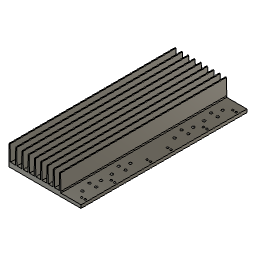
Reproduction Amplifone Deflection Heat Sink (Autodesk Fusion 360 design; units mm, degrees)
Autodesk Fusion 360 part; units mm, degrees
sketch "Sketch1" plane through (0, 0, 0) normal (0, 1, 0) x (1, 0, 0)
  line L0 (-62.23, 0) -> (62.23, 0)
  line L1 (-1.2573, -7.62) -> (1.2573, -7.62) construction
  line L2 (0, -7.62) -> (0, -33.02) construction
  line L3 (-0.762, -33.02) -> (0.762, -33.02)
  line L4 (-1.2573, -7.62) -> (-0.762, -33.02)
  line L5 (1.2573, -7.62) -> (0.762, -33.02)
  line L6 (-51.562, -33.02) -> (-50.038, -33.02)
  line L7 (-49.5427, -7.62) -> (-50.038, -33.02)
  line L8 (-52.0573, -7.62) -> (-51.562, -33.02)
  line L9 (-52.0573, -7.62) -> (-49.5427, -7.62) construction
  line L10 (-50.8, -7.62) -> (-50.8, -33.02) construction
  line L11 (-41.402, -33.02) -> (-39.878, -33.02)
  line L12 (-39.3827, -7.62) -> (-39.878, -33.02)
  line L13 (-41.8973, -7.62) -> (-41.402, -33.02)
  line L14 (-41.8973, -7.62) -> (-39.3827, -7.62) construction
  line L15 (-40.64, -7.62) -> (-40.64, -33.02) construction
  line L16 (-31.242, -33.02) -> (-29.718, -33.02)
  line L17 (-29.2227, -7.62) -> (-29.718, -33.02)
  line L18 (-31.7373, -7.62) -> (-31.242, -33.02)
  line L19 (-31.7373, -7.62) -> (-29.2227, -7.62) construction
  line L20 (-30.48, -7.62) -> (-30.48, -33.02) construction
  line L21 (-21.082, -33.02) -> (-19.558, -33.02)
  line L22 (-19.0627, -7.62) -> (-19.558, -33.02)
  line L23 (-21.5773, -7.62) -> (-21.082, -33.02)
  line L24 (-21.5773, -7.62) -> (-19.0627, -7.62) construction
  line L25 (-20.32, -7.62) -> (-20.32, -33.02) construction
  line L26 (-10.922, -33.02) -> (-9.398, -33.02)
  line L27 (-8.9027, -7.62) -> (-9.398, -33.02)
  line L28 (-11.4173, -7.62) -> (-10.922, -33.02)
  line L29 (-11.4173, -7.62) -> (-8.9027, -7.62) construction
  line L30 (-10.16, -7.62) -> (-10.16, -33.02) construction
  line L31 (9.398, -33.02) -> (10.922, -33.02)
  line L32 (11.4173, -7.62) -> (10.922, -33.02)
  line L33 (8.9027, -7.62) -> (9.398, -33.02)
  line L34 (8.9027, -7.62) -> (11.4173, -7.62) construction
  line L35 (10.16, -7.62) -> (10.16, -33.02) construction
  line L36 (19.558, -33.02) -> (21.082, -33.02)
  line L37 (21.5773, -7.62) -> (21.082, -33.02)
  line L38 (19.0627, -7.62) -> (19.558, -33.02)
  line L39 (19.0627, -7.62) -> (21.5773, -7.62) construction
  line L40 (20.32, -7.62) -> (20.32, -33.02) construction
  line L41 (29.718, -33.02) -> (31.242, -33.02)
  line L42 (31.7373, -7.62) -> (31.242, -33.02)
  line L43 (29.2227, -7.62) -> (29.718, -33.02)
  line L44 (29.2227, -7.62) -> (31.7373, -7.62) construction
  line L45 (30.48, -7.62) -> (30.48, -33.02) construction
  line L46 (39.878, -33.02) -> (41.402, -33.02)
  line L47 (41.8973, -7.62) -> (41.402, -33.02)
  line L48 (39.3827, -7.62) -> (39.878, -33.02)
  line L49 (39.3827, -7.62) -> (41.8973, -7.62) construction
  line L50 (40.64, -7.62) -> (40.64, -33.02) construction
  line L51 (50.038, -33.02) -> (51.562, -33.02)
  line L52 (52.0573, -7.62) -> (51.562, -33.02)
  line L53 (49.5427, -7.62) -> (50.038, -33.02)
  line L54 (49.5427, -7.62) -> (52.0573, -7.62) construction
  line L55 (50.8, -7.62) -> (50.8, -33.02) construction
  line L56 (-62.23, 0) -> (-62.23, -7.62)
  line L57 (62.23, 0) -> (62.23, -7.62)
  line L58 (-62.23, -7.62) -> (-62.23, -33.02)
  line L59 (62.23, -7.62) -> (62.23, -33.02)
  line L60 (-49.5427, -7.62) -> (-41.8973, -7.62)
  line L61 (-39.3827, -7.62) -> (-31.7373, -7.62)
  line L62 (-29.2227, -7.62) -> (-21.5773, -7.62)
  line L63 (-19.0627, -7.62) -> (-11.4173, -7.62)
  line L64 (-8.9027, -7.62) -> (-1.2573, -7.62)
  line L65 (1.2573, -7.62) -> (8.9027, -7.62)
  line L66 (11.4173, -7.62) -> (19.0627, -7.62)
  line L67 (21.5773, -7.62) -> (29.2227, -7.62)
  line L68 (31.7373, -7.62) -> (39.3827, -7.62)
  line L69 (41.8973, -7.62) -> (49.5427, -7.62)
  line L70 (62.23, -33.02) -> (60.706, -33.02)
  line L71 (60.706, -33.02) -> (60.2132, -7.62)
  line L72 (60.2132, -7.62) -> (52.0573, -7.62)
  line L73 (-62.23, -33.02) -> (-60.706, -33.02)
  line L74 (-60.706, -33.02) -> (-60.2132, -7.62)
  line L75 (-60.2132, -7.62) -> (-52.0573, -7.62)
  line L76 (60.2132, -7.62) -> (62.23, -7.62) construction
  line L77 (-60.2132, -7.62) -> (-62.23, -7.62) construction
  dimension "d2" = 124.46
  dimension "d7" = 1.524
  dimension "d8" = 2.5146
  dimension "d10" = 25.4
  dimension "d14" = 10.16
  dimension "d15" = 0
  dimension "d16" = 7.62
  dimension "d17" = 25.4
  dimension "d20" = 2.0168
  dimension "d21" = 1.524
  constraint horizontal L0
  constraint midpoint L0 origin
  constraint horizontal L1
  constraint midpoint L1 L2.start
  constraint horizontal L3
  constraint midpoint L2.end L3
  constraint vertical L2
  constraint coincident origin L2
  constraint perpendicular L9 L56
  constraint perpendicular L54 L57
  constraint equal L56 L57
  constraint parallel L56 L58
  constraint parallel L57 L59
  constraint coincident L57.end L66
  constraint perpendicular L59 L70
  constraint parallel L54 L72
  constraint perpendicular L58 L73
  constraint parallel L9 L75
  constraint equal L76 L77
  constraint equal L70 L73
  constraint equal L58 L59
  measures "d2" distance of L0.start L0.end
  measures "d7" distance of L3.start L3.end
  measures "d8" distance of L1.start L1.end
  measures "d10" vertical distance of L2.start L2.end
  measures "d16" distance of L0.start L56.end
  measures "d17" distance of L56.end L58.end
  measures "d20" distance of L56.end L74.end
  measures "d21" distance of L58.end L73.end
extrude "Extrude1" add sketch "Sketch1" along normal mid plane 268.75
sketch "Sketch2" plane through (0, -134.375, 0) normal (0, -1, 0) x (1, 0, 0)
  line L0 (-62.23, 33.02) -> (-62.23, 0)
  line L1 (-62.23, 0) -> (62.23, 0)
  line L2 (62.23, 0) -> (62.23, 33.02)
  line L3 (62.23, 33.02) -> (60.706, 33.02)
  line L4 (60.706, 33.02) -> (60.2132, 7.62)
  line L5 (60.2132, 7.62) -> (52.0573, 7.62)
  line L6 (52.0573, 7.62) -> (51.562, 33.02)
  line L7 (51.562, 33.02) -> (50.038, 33.02)
  line L8 (50.038, 33.02) -> (49.5427, 7.62)
  line L9 (49.5427, 7.62) -> (41.8973, 7.62)
  line L10 (41.8973, 7.62) -> (41.402, 33.02)
  line L11 (41.402, 33.02) -> (39.878, 33.02)
  line L12 (39.878, 33.02) -> (39.3827, 7.62)
  line L13 (39.3827, 7.62) -> (31.7373, 7.62)
  line L14 (31.7373, 7.62) -> (31.242, 33.02)
  line L15 (31.242, 33.02) -> (29.718, 33.02)
  line L16 (29.718, 33.02) -> (29.2227, 7.62)
  line L17 (29.2227, 7.62) -> (21.5773, 7.62)
  line L18 (21.5773, 7.62) -> (21.082, 33.02)
  line L19 (21.082, 33.02) -> (19.558, 33.02)
  line L20 (19.558, 33.02) -> (19.0627, 7.62)
  line L21 (19.0627, 7.62) -> (11.4173, 7.62)
  line L22 (11.4173, 7.62) -> (10.922, 33.02)
  line L23 (10.922, 33.02) -> (9.398, 33.02)
  line L24 (9.398, 33.02) -> (8.9027, 7.62)
  line L25 (8.9027, 7.62) -> (1.2573, 7.62)
  line L26 (1.2573, 7.62) -> (0.762, 33.02)
  line L27 (0.762, 33.02) -> (-0.762, 33.02)
  line L28 (-0.762, 33.02) -> (-1.2573, 7.62)
  line L29 (-1.2573, 7.62) -> (-8.9027, 7.62)
  line L30 (-8.9027, 7.62) -> (-9.398, 33.02)
  line L31 (-9.398, 33.02) -> (-10.922, 33.02)
  line L32 (-10.922, 33.02) -> (-11.4173, 7.62)
  line L33 (-11.4173, 7.62) -> (-19.0627, 7.62)
  line L34 (-19.0627, 7.62) -> (-19.558, 33.02)
  line L35 (-19.558, 33.02) -> (-21.082, 33.02)
  line L36 (-21.082, 33.02) -> (-21.5773, 7.62)
  line L37 (-21.5773, 7.62) -> (-29.2227, 7.62)
  line L38 (-29.2227, 7.62) -> (-29.718, 33.02)
  line L39 (-29.718, 33.02) -> (-31.242, 33.02)
  line L40 (-31.242, 33.02) -> (-31.7373, 7.62)
  line L41 (-31.7373, 7.62) -> (-39.3827, 7.62)
  line L42 (-39.3827, 7.62) -> (-39.878, 33.02)
  line L43 (-39.878, 33.02) -> (-41.402, 33.02)
  line L44 (-41.402, 33.02) -> (-41.8973, 7.62)
  line L45 (-41.8973, 7.62) -> (-49.5427, 7.62)
  line L46 (-49.5427, 7.62) -> (-50.038, 33.02)
  line L47 (-50.038, 33.02) -> (-51.562, 33.02)
  line L48 (-51.562, 33.02) -> (-52.0573, 7.62)
  line L49 (-52.0573, 7.62) -> (-60.2132, 7.62)
  line L50 (-60.2132, 7.62) -> (-60.706, 33.02)
  line L51 (-60.706, 33.02) -> (-62.23, 33.02)
  line L52 (-62.23, 0) -> (21.5773, 0) construction
  line L53 (21.5773, 0) -> (54.24, 0) construction
  line L54 (54.24, 0) -> (54.24, 5.08) construction
  line L55 (54.24, 5.08) -> (21.5773, 5.08) construction
  line L56 (21.5773, 5.08) -> (21.5773, 0) construction
  line L57 (62.23, 5.08) -> (62.23, 38.1)
  line L58 (62.23, 38.1) -> (21.5773, 38.1)
  line L59 (21.5773, 38.1) -> (21.5773, 5.08)
  line L60 (62.23, 5.08) -> (62.23, 0)
  line L61 (62.23, 0) -> (54.24, 0)
  line L62 (54.24, 0) -> (54.24, 5.08)
  line L63 (62.23, 7.62) -> (62.23, 33.02)
  line L64 (62.23, 0) -> (62.23, 7.62)
  line L65 (21.5773, 5.08) -> (54.24, 5.08)
  line L66 (54.24, 0) -> (62.23, 0)
  line L67 (15.24, 7.62) -> (15.24, 0) construction
  point P0 (-62.23, 7.62)
  point P1 (62.23, 7.62)
  point P2 (60.2132, 7.62)
  point P3 (52.0573, 7.62)
  point P4 (49.5427, 7.62)
  point P5 (41.8973, 7.62)
  point P6 (39.3827, 7.62)
  point P7 (31.7373, 7.62)
  point P8 (29.2227, 7.62)
  dimension "d29" = 5.08
  dimension "d30" = 33.02
  dimension "d79" = 39
  constraint parallel L1 L52
  constraint coincident L0.end L1.start
  constraint horizontal L53
  constraint vertical L54
  constraint horizontal L55
  constraint vertical L56
  constraint vertical L57
  constraint horizontal L58
  constraint vertical L59
  constraint vertical L60
  constraint horizontal L61
  constraint vertical L62
  constraint collinear L57 L63
  constraint collinear L60 L64
  constraint coincident L1.end L2.start
  constraint collinear L61 L66
  constraint coincident L55 L57.start
  constraint coincident L17.end L56
  constraint midpoint L21 L67.start
  constraint coincident L52 L67.end
  constraint vertical L67
  measures "d29" distance of L52.end L55.end
  measures "d30" distance of L55.end L58.end
  measures "d79" distance of L62 L67
extrude "Extrude2" cut sketch "Sketch2" against normal up to surface (268.75 mm away) contours L1 L2 L3 L4 L5 L6 L7 L8 L9 L10 L11 L12 L13 L14 L15 L16 L17 L57 L59 L60 L61 L62 L63 L64 L65 L66
sketch "Sketch3" plane through (0, 0, 5.08) normal (0, 0, 1) x (-1, 0, 0)
  line L0 (-54.24, -134.375) -> (-21.5773, -134.375)
  line L1 (-21.5773, -134.375) -> (-21.5773, 134.375)
  line L2 (-21.5773, 134.375) -> (-54.24, 134.375)
  line L3 (-54.24, 134.375) -> (-54.24, -134.375)
  line L4 (-50.04, 134.375) -> (-50.04, -134.375) construction
  line L5 (-44.34, 134.375) -> (-44.34, -134.375) construction
  line L6 (-41.64, 134.375) -> (-41.64, -134.375) construction
  line L7 (-36.24, 134.375) -> (-36.24, -134.375) construction
  line L8 (-30.74, 134.375) -> (-30.74, -134.375) construction
  line L9 (-15.24, 134.375) -> (-15.24, -134.375) construction
  line L10 (-54.24, -134.375) -> (-21.5773, -134.375)
  line L11 (-21.5773, -134.375) -> (-21.5773, 134.375)
  line L12 (-21.5773, 134.375) -> (-54.24, 134.375)
  line L13 (-54.24, 134.375) -> (-54.24, -134.375)
  circle A0 centre (-50.04, 123.375) radius 1.6
  circle A1 centre (-50.04, 75.575) radius 1.6
  circle A2 centre (-50.04, 17.575) radius 1.6
  circle A3 centre (-50.04, -15.925) radius 1.6
  circle A4 centre (-50.04, -73.825) radius 1.6
  circle A5 centre (-50.04, -121.325) radius 1.6
  circle A6 centre (-44.34, 123.375) radius 1.6
  circle A7 centre (-44.34, 75.575) radius 1.6
  circle A8 centre (-44.34, 17.575) radius 1.6
  circle A9 centre (-44.34, -15.925) radius 1.6
  circle A10 centre (-44.34, -73.825) radius 1.6
  circle A11 centre (-44.34, -121.325) radius 1.6
  line L14 (-50.04, 123.375) -> (-44.34, 123.375) construction
  line L15 (-50.04, 75.575) -> (-44.34, 75.575) construction
  line L16 (-50.04, 17.575) -> (-44.34, 17.575) construction
  line L17 (-50.04, -15.925) -> (-44.34, -15.925) construction
  line L18 (-50.04, -73.825) -> (-44.34, -73.825) construction
  line L19 (-50.04, -121.325) -> (-44.34, -121.325) construction
  line L20 (-30.74, 97.175) -> (-41.64, 97.175) construction
  line L21 (-30.74, 49.575) -> (-41.64, 49.575) construction
  line L22 (-30.74, -52.225) -> (-41.64, -52.225) construction
  line L23 (-30.74, -99.825) -> (-41.64, -99.825) construction
  circle A12 centre (-41.64, 97.175) radius 2
  circle A13 centre (-30.74, 49.575) radius 2
  circle A14 centre (-30.74, -52.225) radius 2
  circle A15 centre (-30.74, -99.825) radius 2
  circle A16 centre (-30.74, 97.175) radius 2
  circle A17 centre (-41.64, 49.575) radius 2
  circle A18 centre (-41.64, -52.225) radius 2
  circle A19 centre (-41.64, -99.825) radius 2
  circle A20 centre (-36.24, 113.975) radius 2.1
  circle A21 centre (-36.24, 83.875) radius 2.1
  circle A22 centre (-36.24, 66.375) radius 2.1
  circle A23 centre (-36.24, 36.275) radius 2.1
  circle A24 centre (-36.24, -35.325) radius 2.1
  circle A25 centre (-36.24, -65.425) radius 2.1
  circle A26 centre (-15.24, 123.175) radius 2.1
  circle A27 centre (-15.24, -121.225) radius 2.1
  circle A28 centre (-36.24, -83.025) radius 2.1
  circle A29 centre (-36.24, -113.125) radius 2.1
  point P0 (62.23, 134.375)
  dimension "d73" = 4.2
  dimension "d74" = 9.9
  dimension "d75" = 12.6
  dimension "d76" = 18
  dimension "d77" = 23.5
  dimension "d78" = 39
  dimension "d87" = 3.2
  dimension "d94" = 11
  dimension "d95" = 58.8
  dimension "d96" = 116.8
  dimension "d97" = 150.3
  dimension "d98" = 208.2
  dimension "d99" = 255.7
  dimension "d100" = 37.2
  dimension "d101" = 84.8
  dimension "d102" = 186.6
  dimension "d103" = 234.2
  dimension "d104" = 4
  dimension "d105" = 4.2
  dimension "d106" = 20.4
  dimension "d107" = 50.5
  dimension "d108" = 68
  dimension "d109" = 98.1
  dimension "d110" = 169.7
  dimension "d111" = 199.8
  dimension "d112" = 217.4
  dimension "d113" = 247.5
  dimension "d114" = 11.2
  dimension "d115" = 255.6
  dimension "d116" = 4.2
  dimension "d117" = 4
  dimension "d118" = 3.2
  constraint coincident L2 L4.start
  constraint coincident L0 L4.end
  constraint perpendicular L0 L4
  constraint coincident L2 L5.start
  constraint coincident L0 L5.end
  constraint perpendicular L0 L5
  constraint coincident L2 L6.start
  constraint coincident L0 L6.end
  constraint perpendicular L0 L6
  constraint coincident L2 L7.start
  constraint coincident L0 L7.end
  constraint perpendicular L0 L7
  constraint coincident L2 L8.start
  constraint coincident L0 L8.end
  constraint perpendicular L0 L8
  constraint coincident L2 L9.start
  constraint coincident L0 L9.end
  constraint perpendicular L0 L9
  constraint coincident L4 A0.centre
  constraint coincident L4 A5.centre
  constraint coincident L4 A4.centre
  constraint coincident L4 A3.centre
  constraint coincident L4 A2.centre
  constraint coincident L4 A1.centre
  constraint coincident A0.centre L14.start
  constraint coincident L5 A6.centre
  constraint perpendicular L5 L14
  constraint coincident A1.centre L15.start
  constraint coincident L5 A7.centre
  constraint perpendicular L5 L15
  constraint coincident A2.centre L16.start
  constraint coincident L5 A8.centre
  constraint perpendicular L5 L16
  constraint coincident A3.centre L17.start
  constraint coincident L5 A9.centre
  constraint perpendicular L5 L17
  constraint coincident A4.centre L18.start
  constraint coincident L5 A10.centre
  constraint perpendicular L5 L18
  constraint coincident A5.centre L19.start
  constraint coincident L5 A11.centre
  constraint perpendicular L5 L19
  constraint coincident A6.centre L14.end
  constraint coincident A7.centre L15.end
  constraint coincident A8.centre L16.end
  constraint coincident A9.centre L17.end
  constraint coincident A10.centre L18.end
  constraint coincident A11.centre L19.end
  constraint coincident L8 L20.start
  constraint coincident L6 L20.end
  constraint perpendicular L6 L20
  constraint coincident L8 L21.start
  constraint coincident L6 L21.end
  constraint perpendicular L6 L21
  constraint coincident L8 L22.start
  constraint coincident L6 L22.end
  constraint perpendicular L6 L22
  constraint coincident L8 L23.start
  constraint coincident L6 L23.end
  constraint perpendicular L6 L23
  constraint coincident L20.end A12.centre
  constraint coincident L20.start A16.centre
  constraint coincident L21.end A17.centre
  constraint coincident L21.start A13.centre
  constraint coincident L22.end A18.centre
  constraint coincident L22.start A14.centre
  constraint coincident L23.end A19.centre
  constraint coincident L23.start A15.centre
  constraint coincident L9 A26.centre
  constraint coincident L9 A27.centre
  constraint coincident L7 A20.centre
  constraint coincident L7 A21.centre
  constraint coincident L7 A22.centre
  constraint coincident L7 A23.centre
  constraint coincident L7 A24.centre
  constraint coincident L7 A25.centre
  constraint coincident L7 A28.centre
  constraint coincident L7 A29.centre
  constraint equal A26 A27
  constraint equal A12 A17
  constraint equal A17 A18
  constraint equal A18 A19
  constraint equal A13 A16
  constraint equal A13 A14
  constraint equal A14 A15
  constraint equal A20 A21
  constraint equal A21 A22
  constraint equal A22 A23
  constraint equal A23 A24
  constraint equal A24 A25
  constraint equal A25 A28
  constraint equal A28 A29
  constraint equal A0 A1
  constraint equal A1 A2
  constraint equal A2 A3
  constraint equal A3 A4
  constraint equal A4 A5
  constraint equal A6 A7
  constraint equal A7 A8
  constraint equal A8 A9
  constraint equal A9 A10
  constraint equal A10 A11
  measures "d73" distance of L3 L4
  measures "d74" distance of L3 L5
  measures "d75" distance of L3 L6
  measures "d76" distance of L3 L7
  measures "d77" distance of L3 L8
  measures "d78" distance of L3 L9
  measures "d87" diameter of A0
  measures "d94" distance of L2 L14
  measures "d95" distance of L2 L15
  measures "d96" distance of L2 L16
  measures "d97" distance of L2 L17
  measures "d98" distance of L2 L18
  measures "d99" distance of L2 L19
  measures "d100" distance of L2 L20
  measures "d101" distance of L2 L21
  measures "d102" distance of L2 L22
  measures "d103" distance of L2 L23
  measures "d104" diameter of A12
  measures "d105" diameter of A20
  measures "d106" distance of L2 A20.centre
  measures "d107" distance of L2 A21.centre
  measures "d108" distance of L2 A22.centre
  measures "d109" distance of L2 A23.centre
  measures "d110" distance of L2 A24.centre
  measures "d111" distance of L2 A25.centre
  measures "d112" distance of L2 A28.centre
  measures "d113" distance of L2 A29.centre
  measures "d114" distance of L9.start A26.centre
  measures "d115" distance of L9.start A27.centre
  measures "d116" diameter of A26
  measures "d117" diameter of A16
  measures "d118" diameter of A6
hole "Hole1" at (50.04, -123.375, 5.08) at (50.04, -75.575, 5.08) at (50.04, -17.575, 5.08) at (50.04, 15.925, 5.08) at (50.04, 73.825, 5.08) at (50.04, 121.325, 5.08) direction (0, 0, -1) diameter 3.2 end through all
hole "Hole2" at (44.34, -123.375, 5.08) at (44.34, -75.575, 5.08) at (44.34, -17.575, 5.08) at (44.34, 15.925, 5.08) at (44.34, 73.825, 5.08) at (44.34, 121.325, 5.08) direction (0, 0, -1) diameter 3.2 end through all
hole "Hole3" at (41.64, -97.175, 5.08) at (41.64, -49.575, 5.08) at (41.64, 52.225, 5.08) at (41.64, 99.825, 5.08) direction (0, 0, -1) diameter 4 end through all
hole "Hole4" at (36.24, -113.975, 5.08) at (36.24, -83.875, 5.08) at (36.24, -66.375, 5.08) at (36.24, -36.275, 5.08) at (36.24, 35.325, 5.08) at (36.24, 65.425, 5.08) at (36.24, 83.025, 5.08) at (36.24, 113.125, 5.08) direction (0, 0, -1) diameter 4.2 end through all
hole "Hole5" at (30.74, -97.175, 5.08) at (30.74, -49.575, 5.08) at (30.74, 52.225, 5.08) at (30.74, 99.825, 5.08) direction (0, 0, -1) diameter 4 end through all
sketch "Sketch4" plane through (0, 0, 7.62) normal (0, 0, 1) x (-1, 0, 0)
  line L0 (-19.0627, 134.375) -> (-19.0627, -134.375)
  line L1 (-19.0627, -134.375) -> (-11.4173, -134.375)
  line L2 (-11.4173, -134.375) -> (-11.4173, 134.375)
  line L3 (-11.4173, 134.375) -> (-19.0627, 134.375)
  point P0 (-15.24, 123.175)
  point P1 (-15.24, -121.225)
  point P2 (-15.24, 123.175)
  point P3 (-15.24, -121.225)
  constraint coincident P2 P0
  constraint coincident P3 P1
hole "Hole7" at (15.24, -123.175, 7.62) at (15.24, 121.225, 7.62) direction (0, 0, -1) diameter 4.2 end through all
hole "Hole6" at (15.24, -123.175, 5.08) at (15.24, 121.225, 5.08) direction (0, 0, -1) diameter 4.2 depth 5.08 tip angle 118
extrude "Extrude3" cut sketch "Sketch3" along normal up to surface (2.54 mm away) and the other way up to surface (5.08 mm away) contours A0 | A1 | A2 | A3 | A4 | A5 | A6 | A7 | A8 | A9 | A10 | A11 | A12 | A13 | A14 | A15 | A16 | A17 | A18 | A19 | A20 | A21 | A22 | A23 | A24 | A25 | A26 | A27 | A28 | A29
equation "ProfileWidth = 4.9 in"
equation "d2 = ProfileWidth"
equation "BaseThickness = 0.3 in"
equation "FinWidthTip = 0.06 in"
equation "FinWidthBase = 0.099 in"
equation "d7 = FinWidthTip"
equation "d8 = FinWidthBase"
equation "FinLength = 1 in"
equation "d10 = FinLength"
equation "FinSpacing = 0.4 in"
equation "d14 = FinSpacing"
equation "d16 = BaseThickness"
equation "d17 = FinLength"
equation "EndFinWidthBase = 0.0794 in"
equation "d20 = EndFinWidthBase"
equation "d21 = FinWidthTip"
equation "HeatsinkKeepWidth = 81.9 mm"
equation "FlatHeight = 0.2 in"
equation "FlatDepth = 32.90 mm"
equation "d29 = FlatHeight"
equation "d30 = BaseThickness + FinLength"
equation "DezRow1 = 4.2 mm"
equation "DezRow2 = 9.9 mm"
equation "DezRow3 = 12.6 mm"
equation "DezRow4 = 18 mm"
equation "DezRow5 = 23.5 mm"
equation "DezRow6 = 39 mm"
equation "Dez1Left = 11 mm"
equation "Dez2Left = 58.8 mm"
equation "Dez3Left = 116.8 mm"
equation "Dez4Left = 150.3 mm"
equation "Dez5Left = 208.2 mm"
equation "Dez6Left = 255.7 mm"
equation "Dez7ALeft = 11.2 mm"
equation "Dez7BLeft = 255.6 mm"
equation "Dez8ALeft = 20.4 mm"
equation "Dez8BLeft = 50.5 mm"
equation "Dez9ALeft = 68.0 mm"
equation "Dez9BLeft = 98.1 mm"
equation "Dez10ALeft = 169.7 mm"
equation "Dez10BLeft = 199.8 mm"
equation "Dez11ALeft = 217.4 mm"
equation "Dez11BLeft = 247.5 mm"
equation "Dez12Left = 37.2 mm"
equation "Dez13Left = 84.8 mm"
equation "Dez14Left = 186.6 mm"
equation "Dez15Left = 234.2 mm"
equation "d73 = DezRow1"
equation "d74 = DezRow2"
equation "d75 = DezRow3"
equation "d76 = DezRow4"
equation "d77 = DezRow5"
equation "d78 = DezRow6"
equation "d79 = DezRow6"
equation "DezRow1Diameter = 3.2 mm"
equation "DezRow2Diameter = DezRow1Diameter"
equation "DezRow3Diameter = 4 mm"
equation "DezRow4Diameter = 4.2 mm"
equation "DezRow5Diameter = DezRow3Diameter"
equation "DezRow6Diameter = 4.2 mm"
equation "d87 = DezRow1Diameter"
equation "d94 = Dez1Left"
equation "d95 = Dez2Left"
equation "d96 = Dez3Left"
equation "d97 = Dez4Left"
equation "d98 = Dez5Left"
equation "d99 = Dez6Left"
equation "d100 = Dez12Left"
equation "d101 = Dez13Left"
equation "d102 = Dez14Left"
equation "d103 = Dez15Left"
equation "d104 = DezRow3Diameter"
equation "d105 = DezRow4Diameter"
equation "d106 = Dez8ALeft"
equation "d107 = Dez8BLeft"
equation "d108 = Dez9ALeft"
equation "d109 = Dez9BLeft"
equation "d110 = Dez10ALeft"
equation "d111 = Dez10BLeft"
equation "d112 = Dez11ALeft"
equation "d113 = Dez11BLeft"
equation "d114 = Dez7ALeft"
equation "d115 = Dez7BLeft"
equation "d116 = DezRow6Diameter"
equation "d117 = DezRow5Diameter"
equation "d118 = DezRow2Diameter"
equation "d123 = DezRow1Diameter"
equation "d125 = DezRow2Diameter"
equation "d127 = DezRow3Diameter"
equation "d129 = DezRow4Diameter"
equation "d131 = DezRow5Diameter"
equation "d133 = DezRow6Diameter"
equation "d136 = DezRow6Diameter"
